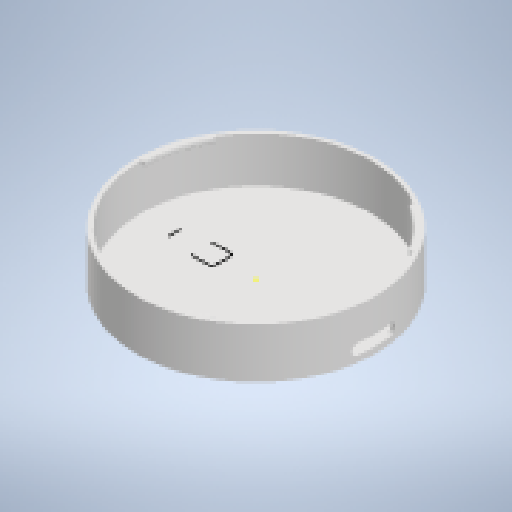
# Autodesk Inventor part: bottom_basket
Saved by Autodesk Inventor 2023 (Build 270158000, 158)
## iProperties
Created: 2025-12-29
Part Number: bottom_basket
Material: Generic
Document SubType Name: Modeling
Designer: Justin Pascual
Density: 1 g/cm^3
Appearance: Default
Author: Justin Pascual
Autodesk Inventor part; units mm, degrees
ref_plane "YZ Plane" through (0, 0, 0) normal (1, 0, 0) x (0, 1, 0)
ref_plane "XZ Plane" through (0, 0, 0) normal (0, 1, 0) x (-1, 0, 0)
ref_plane "XY Plane" through (0, 0, 0) normal (0, 0, 1) x (1, 0, 0)
sketch "Sketch1" plane through (0, 0, 0) normal (0, 1, 0) x (-1, 0, 0)
  circle A0 centre (0, 0) radius 69.85
  dimension "d0" = 139.7
  constraints: 1 centre point, 1 coincident
  measures "d0" diameter of A0
extrude "Extrusion1" add sketch "Sketch1" along normal blind 29.21
sketch "Sketch3" plane through (0, 29.21, 0) normal (0, 1, 0) x (1, 0, 0)
  circle A0 centre (0, 0) radius 67.31
  dimension "d5" = 134.62
  constraints: 1 centre point, 1 coincident
  measures "d5" diameter of A0
extrude "Extrusion2" cut sketch "Sketch3" against normal blind 26.67
sketch "Sketch6" plane through (0, 0, 0) normal (1, 0, 0) x (0, 1, 0)
  line L0 (29.21, 67.31) -> (2.54, 67.31) projected
  line L1 (29.21, 67.31) -> (26.924, 67.31)
  line L2 (26.924, 67.31) -> (26.924, 65.024)
  line L3 (26.924, 65.024) -> (29.21, 65.024)
  line L4 (29.21, 65.024) -> (29.21, 67.31)
  line L5 (-5.842, 0) -> (35.052, 0) projected
  line L6 (29.21, -69.85) -> (29.21, 69.85) projected
  point P0 (0, 0)
  dimension "d21" = 2.286
  dimension "d22" = 2.286
  dimension "d36" = 0
  constraints: 8 end point, 2 parallel, 1 horizontal, 1 perpendicular, 1 point on line
  measures "d21" distance of L3.end L2.end
  measures "d22" distance of L2.end L1.end
  measures "d36" distance between parallel lines of L6 L4
revolve "Revolution1" add sketch "Sketch6" angle 30 about axis through (0, -10, 0) along (0, 1, 0)
fillet "Fillet2" radius 1.143 2 edges at (16.8294, 26.924, 62.8084) (16.8294, 29.21, 62.8084)
fillet "Fillet3" radius 1.143 5 edges at (32.6794, 28.8753, 56.6023) (32.512, 28.067, 56.3124) (32.6794, 27.2587, 56.6023) (33.3692, 29.21, 57.7972) (33.3692, 26.924, 57.7972)
pattern_circular "Circular Pattern1" count 3 over 360 about axis through (0, 0, 0) along (0, 1, 0) of "Revolution1", "Fillet2", "Fillet3"
sketch "Sketch9" plane through (0, 0, 0) normal (1, 0, 0) x (0, 1, 0)
  circle A0 centre (6.8717, 0) radius 3.175 construction
  line L0 (6.8717, 0) -> (6.8717, -12.7) construction
  line L1 (6.8717, 0) -> (6.8717, 12.7) construction
  line L2 (6.8717, -12.7) -> (6.8717, -12.7)
  line L3 (3.6967, -9.525) -> (3.6967, 9.525)
  line L4 (6.8717, 12.7) -> (6.8717, 12.7)
  line L5 (10.0467, 9.525) -> (10.0467, -9.525)
  arc A1 (6.8717, -12.7) -> (10.0467, -9.525) centre (6.8717, -9.525) ccw
  arc A2 (3.6967, -9.525) -> (6.8717, -12.7) centre (6.8717, -9.525) ccw
  arc A3 (6.8717, 12.7) -> (3.6967, 9.525) centre (6.8717, 9.525) ccw
  arc A4 (10.0467, 9.525) -> (6.8717, 12.7) centre (6.8717, 9.525) ccw
  point P0 (0, 0)
  dimension "d37" = 6.35
  dimension "d48" = 12.7
  dimension "d49" = 12.7
  dimension "d50" = 3.175
  constraints: 12 end point, 8 point on circle, 8 tangent, 5 centre point, 3 equal radius, 2 parallel, 1 horizontal, 1 perpendicular, 1 point on line, 1 vertical
  measures "d37" diameter of A0
  measures "d48" distance of L0.start L0.end
  measures "d49" distance of L0.start L1.end
  measures "d50" radius of A1
extrude "Extrusion9" cut sketch "Sketch9" along normal through all
sketch "Sketch15" plane through (0, 2.54, 0) normal (0, 1, 0) x (1, 0, 0)
  line L0 (-19.7435, -6.1595) -> (-19.7435, 6.1595)
  line L1 (-31.8085, -6.1595) -> (-19.7435, -6.1595)
  line L2 (-31.8085, 6.1595) -> (-19.7435, 6.1595)
  line L3 (-47.8867, -3.627) -> (-47.8867, 3.627)
  point P0 (0, 0)
  constraints: 8 end point, 2 horizontal, 2 vertical, 6 other
sketch "Sketch16" plane through (0, 2.54, 0) normal (0, 1, 0) x (1, 0, 0)
  line L0 (-19.7435, -6.1595) -> (-19.7435, 6.1595) construction
  line L1 (-31.8085, 6.1595) -> (-19.7435, 6.1595) construction
  line L2 (-31.8085, -6.1595) -> (-19.7435, -6.1595) construction
  line L3 (-47.8867, -3.627) -> (-47.8867, 3.627) construction
  line L4 (-19.7435, 0) -> (-19.7435, 15.24)
  line L5 (-19.7435, 15.24) -> (-45.1435, 15.24)
  line L6 (-19.7435, 0) -> (-19.7435, -15.24)
  line L7 (-19.7435, -15.24) -> (-45.1435, -15.24)
  line L8 (-45.1435, -15.24) -> (-45.1435, 15.24)
  point P0 (0, 0)
  dimension "d53" = 15.24
  dimension "d54" = 25.4
  dimension "d55" = 15.24
  dimension "d56" = 25.4
  constraints: 10 end point, 2 perpendicular, 1 midpoint, 1 point on line, 1 vertical
  measures "d53" distance of L4.start L4.end
  measures "d54" distance of L4.end L5.end
  measures "d55" distance of L4.start L6.end
  measures "d56" distance of L6.end L7.end
extrude "Extrusion10" add sketch "Sketch16" along normal blind 13.589
sketch "Sketch17" plane through (0, 16.129, 0) normal (0, 1, 0) x (1, 0, 0)
  circle A0 centre (-38.7935, -11.43) radius 2.159
  circle A1 centre (-38.7935, 11.43) radius 2.159
  line L0 (-45.1435, -15.24) -> (-19.7435, -15.24) projected
  line L1 (-45.1435, 15.24) -> (-45.1435, -15.24) projected
  point P0 (0, 0)
  dimension "d59" = 4.318
  dimension "d60" = 4.318
  dimension "d61" = 22.86
  dimension "d62" = 3.81
  dimension "d63" = 6.35
  dimension "d64" = 6.35
  constraints: 2 centre point
  measures "d59" diameter of A0
  measures "d60" diameter of A1
  measures "d61" distance of A0.centre A1.centre
  measures "d62" distance from line of L0 A0.centre
  measures "d63" distance from line of L1 A1.centre
  measures "d64" distance from line of L1 A0.centre
extrude "Extrusion11" cut sketch "Sketch17" against normal blind 13.589
sketch "Sketch18" plane through (0, 2.54, 0) normal (0, 1, 0) x (1, 0, 0)
  circle A0 centre (0, 0) radius 3.81
  dimension "d67" = 7.62
  constraints: 1 centre point, 1 coincident
  measures "d67" diameter of A0
extrude "Extrusion12" cut sketch "Sketch18" against normal blind 0.635
body "Solid1"
